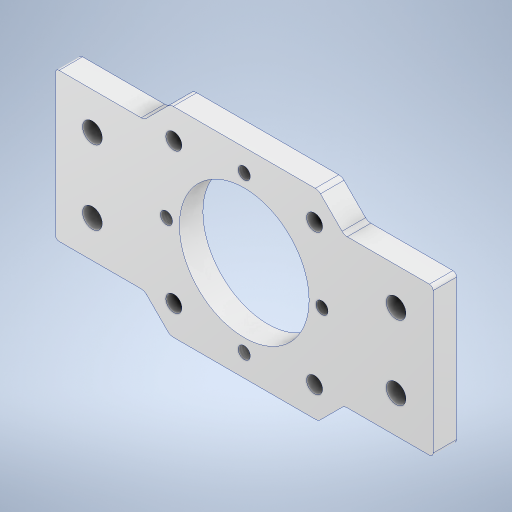
# Autodesk Inventor part: Z-Axis Motor Plate
Saved by Autodesk Inventor 2024 (Build 280153000, 153)
## iProperties
Created: 2024-08-01
Part Number: Z-Axis Motor Plate
Material: Aluminum 6061
Document SubType Name: Modeling
Designer: Ishaan
Density: 2.7 g/cm^3
Appearance: Aluminum - Flat
Author: Ishaan
Autodesk Inventor part; units mm, degrees
ref_plane "YZ Plane" through (0, 0, 0) normal (1, 0, 0) x (0, 1, 0)
ref_plane "XZ Plane" through (0, 0, 0) normal (0, 1, 0) x (-1, 0, 0)
ref_plane "XY Plane" through (0, 0, 0) normal (0, 0, 1) x (1, 0, 0)
sketch "Sketch1" plane through (0, 0, 0) normal (0, 0, 1) x (1, 0, 0)
  line L0 (51, -20) -> (-51, -20)
  line L1 (-51, -20) -> (-51, 20)
  line L2 (-51, 20) -> (51, 20)
  line L3 (51, 20) -> (51, -20)
  line L4 (51, -20) -> (-51, 20) construction
  line L5 (-51, -20) -> (51, 20) construction
  line L6 (21, -21) -> (-21, -21) construction
  line L7 (-21, -21) -> (-21, 21) construction
  line L8 (-21, 21) -> (21, 21) construction
  line L9 (21, 21) -> (21, -21) construction
  line L10 (21, -21) -> (-21, 21) construction
  line L11 (-21, -21) -> (21, 21) construction
  line L12 (29.6985, 0) -> (0, 29.6985) construction
  line L13 (0, 29.6985) -> (-29.6985, 0) construction
  line L14 (-29.6985, 0) -> (0, -29.6985) construction
  line L15 (0, -29.6985) -> (29.6985, 0) construction
  line L16 (29.6985, 0) -> (-29.6985, 0) construction
  line L17 (0, 29.6985) -> (0, -29.6985) construction
  circle A0 centre (0, 0) radius 26 construction
  line L18 (20, -27) -> (-20, -27)
  line L19 (-27, -20) -> (-27, 20)
  line L20 (-20, 27) -> (20, 27)
  line L21 (27, 20) -> (27, -20)
  line L22 (27, -27) -> (-27, 27) construction
  line L23 (-27, -27) -> (27, 27) construction
  line L24 (24.4641, -27) -> (17.5359, -27)
  line L25 (-27, 20) -> (-20, 27)
  line L26 (20, 27) -> (27, 20)
  line L27 (20, -27) -> (27, -20)
  line L28 (-20, -27) -> (-27, -20)
  circle A1 centre (-21, 21) radius 3.5355
  point P0 (28.5056, -20)
  point P1 (27, 20)
  point P2 (27, -20)
  point P3 (27, 20)
  point P4 (-27, -20)
  point P5 (27, -20)
  point P6 (-27, -20)
  dimension "d0" = 102
  dimension "d1" = 40
  dimension "d2" = 42
  dimension "d3" = 42
  dimension "d4" = 42
  dimension "d5" = 42
  dimension "d6" = 52
  dimension "d8" = 54
  dimension "d43" = 7
  dimension "d44" = 7
  dimension "d45" = 7
  dimension "d46" = 7
  dimension "d47" = 7
  dimension "d48" = 7
  dimension "d49" = 7
  dimension "d50" = 7
  dimension "d51" = 7
  dimension "d52" = 6
  dimension "d53" = 6
  constraints: 58 end point, 9 point on line, 8 midpoint, 8 parallel, 4 perpendicular, 3 horizontal, 2 centre point, 2 coincident, 1 collinear, 1 tangent, 1 vertical
  measures "d0" distance of L1.end L2.end
  measures "d1" distance of L0.end L1.end
  measures "d2" distance of L7.end L8.end
  measures "d3" distance of L6.end L7.end
  measures "d4" distance of L13.end L12.end
  measures "d5" distance of L12.start L12.end
  measures "d6" diameter of A0
  measures "d8" distance of L23.start L22.end
  measures "d43" distance between parallel lines of L20 L2
  measures "d44" distance of L19.end L22.end
  measures "d45" distance of L20.start L22.end
  measures "d46" distance of L20.end L23.end
  measures "d47" distance of L21.start L23.end
  measures "d48" distance of L18.start L22.start
  measures "d49" distance of L21.end L22.start
  measures "d50" distance of L18.end L23.start
  measures "d51" distance of L19.start L23.start
  measures "d52" distance from line of L20 L7.end
  measures "d53" distance from line of L7.end L19
extrude "Extrusion1" add sketch "Sketch1" along normal blind 6.35
fillet "Fillet1" radius 1 4 edges at (-51, 20, 3.175) (-51, -20, 3.175) (51, 20, 3.175) (51, -20, 3.175)
fillet "Fillet2" radius 2 8 edges at (-20, -27, 3.175) (-20, 27, 3.175) (20, 27, 3.175) (20, -27, 3.175) (-27, -20, 3.175) (-27, 20, 3.175) (27, -20, 3.175) (27, 20, 3.175)
sketch "Sketch2" plane through (0, 0, 6.35) normal (0, 0, 1) x (1, 0, 0)
  circle A0 centre (0, 0) radius 17.5
  dimension "d13" = 35
  constraints: 1 centre point, 1 coincident
  measures "d13" diameter of A0
extrude "Extrusion2" cut sketch "Sketch2" against normal through all
sketch "Sketch3" plane through (0, 0, 6.35) normal (0, 0, 1) x (1, 0, 0)
  circle A0 centre (0, 0) radius 21 construction
  circle A1 centre (0, 0) radius 17.5 projected
  line L0 (0, -21) -> (21, 0) construction
  line L1 (21, 0) -> (0, 21) construction
  line L2 (0, 21) -> (-21, 0) construction
  line L3 (-21, 0) -> (0, -21) construction
  line L4 (0, -21) -> (0, 21) construction
  line L5 (21, 0) -> (-21, 0) construction
  dimension "d17" = 42
  constraints: 12 end point, 5 coincident, 2 midpoint, 2 parallel, 2 perpendicular, 1 horizontal, 1 horizontal alignment, 2 other
hole "Hole1" at (0, 21, 6.35) at (21, 0, 6.35) at (0, -21, 6.35) at (-21, 0, 6.35) direction (0, 0, -1) diameter 3.242 end through all thread size "M4x0.7" class "6H" standard "ANSI Metric M Profile"
sketch "Sketch4" plane through (0, 0, 6.35) normal (0, 0, 1) x (1, 0, 0)
  line L0 (41, -10) -> (-41, -10)
  line L1 (-41, -10) -> (-41, 10)
  line L2 (-41, 10) -> (41, 10)
  line L3 (41, 10) -> (41, -10)
  line L4 (41, -10) -> (-41, 10) construction
  line L5 (-41, -10) -> (41, 10) construction
  line L6 (-51, 19) -> (-51, -19) projected
  point P0 (0, 0)
  dimension "d25" = 20
  dimension "d26" = 10
  constraints: 12 end point, 4 coincident, 2 midpoint, 2 parallel, 1 horizontal, 1 perpendicular
  measures "d25" distance of L0.end L1.end
  measures "d26" distance between parallel lines of L1 L6
hole "Hole2" at (-41, 10, 6.35) at (-41, -10, 6.35) at (41, 10, 6.35) at (41, -10, 6.35) direction (0, 0, -1) diameter 5.3 end through all
sketch "Sketch5" plane through (0, 0, 6.35) normal (0, 0, 1) x (1, 0, 0)
  line L0 (19, -19) -> (-19, -19)
  line L1 (-19, -19) -> (-19, 19)
  line L2 (-19, 19) -> (19, 19)
  line L3 (19, 19) -> (19, -19)
  line L4 (19, -19) -> (-19, 19) construction
  line L5 (-19, -19) -> (19, 19) construction
  point P0 (0, 0)
  dimension "d34" = 38
  dimension "d35" = 38
  constraints: 12 end point, 4 coincident, 2 midpoint, 2 parallel, 1 horizontal, 1 perpendicular
  measures "d34" distance of L1.end L2.end
  measures "d35" distance of L0.end L1.end
hole "Hole3" at (-19, 19, 6.35) at (19, 19, 6.35) at (19, -19, 6.35) at (-19, -19, 6.35) direction (0, 0, -1) diameter 4.3 end through all
equation "\"d44\" = d43"
equation "\"d45\" = d44"
equation "\"d46\" = d44"
equation "\"d47\" = d46"
equation "\"d48\" = d44"
equation "\"d49\" = d48"
equation "\"d50\" = d44"
equation "\"d51\" = d50"
equation "\"d53\" = d52"
body "Solid1"
